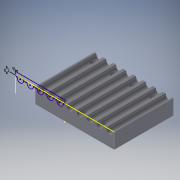
# Autodesk Inventor part: belt-clamp-15mm-htd
Saved by Autodesk Inventor 2016 (Build 200138000, 138)
## iProperties
Created: 2015-10-25
Part Number: belt-clamp-15mm-htd
Material: Generic
Document SubType Name: Modeling
Designer: as
Density: 1 g/cm^3
Appearance: Default
Author: as
Autodesk Inventor part; units mm, degrees
ref_plane "YZ Plane" through (0, 0, 0) normal (1, 0, 0) x (0, 1, 0)
ref_plane "XZ Plane" through (0, 0, 0) normal (0, 1, 0) x (-1, 0, 0)
ref_plane "XY Plane" through (0, 0, 0) normal (0, 0, 1) x (1, 0, 0)
sketch "HTD 5m profile" plane through (0, 0, 0) normal (0, 0, 1) x (1, 0, 0)
  arc A0 (5.5026, 4.809) -> (5.0726, 4.379) centre (5.5026, 4.379) ccw
  line L0 (5.0726, 4.379) -> (5.0726, 4.229)
  arc A1 (3.5726, 2.729) -> (5.0726, 4.229) centre (3.5726, 4.229) ccw
  line L1 (3.5726, 2.729) -> (3.4726, 2.729)
  arc A2 (1.9726, 4.229) -> (3.4726, 2.729) centre (3.4726, 4.229) ccw
  line L2 (1.9726, 4.229) -> (1.9726, 4.379)
  arc A3 (1.9726, 4.379) -> (1.5426, 4.809) centre (1.5426, 4.379) ccw
  line L3 (1.5426, 4.809) -> (0.9326, 4.809)
  line L4 (0.9326, 4.809) -> (0.9326, 6.539)
  line L5 (6.5426, 4.809) -> (5.5026, 4.809)
  arc A4 (10.5026, 4.809) -> (10.0726, 4.379) centre (10.5026, 4.379) ccw
  line L6 (10.0726, 4.379) -> (10.0726, 4.229)
  arc A5 (8.5726, 2.729) -> (10.0726, 4.229) centre (8.5726, 4.229) ccw
  line L7 (8.5726, 2.729) -> (8.4726, 2.729)
  arc A6 (6.9726, 4.229) -> (8.4726, 2.729) centre (8.4726, 4.229) ccw
  line L8 (6.9726, 4.229) -> (6.9726, 4.379)
  arc A7 (6.9726, 4.379) -> (6.5426, 4.809) centre (6.5426, 4.379) ccw
  line L9 (11.5426, 4.809) -> (10.5026, 4.809)
  arc A8 (15.5026, 4.809) -> (15.0726, 4.379) centre (15.5026, 4.379) ccw
  line L10 (15.0726, 4.379) -> (15.0726, 4.229)
  arc A9 (13.5726, 2.729) -> (15.0726, 4.229) centre (13.5726, 4.229) ccw
  line L11 (13.5726, 2.729) -> (13.4726, 2.729)
  arc A10 (11.9726, 4.229) -> (13.4726, 2.729) centre (13.4726, 4.229) ccw
  line L12 (11.9726, 4.229) -> (11.9726, 4.379)
  arc A11 (11.9726, 4.379) -> (11.5426, 4.809) centre (11.5426, 4.379) ccw
  line L13 (16.5426, 4.809) -> (15.5026, 4.809)
  arc A12 (20.5026, 4.809) -> (20.0726, 4.379) centre (20.5026, 4.379) ccw
  line L14 (20.0726, 4.379) -> (20.0726, 4.229)
  arc A13 (18.5726, 2.729) -> (20.0726, 4.229) centre (18.5726, 4.229) ccw
  line L15 (18.5726, 2.729) -> (18.4726, 2.729)
  arc A14 (16.9726, 4.229) -> (18.4726, 2.729) centre (18.4726, 4.229) ccw
  line L16 (16.9726, 4.229) -> (16.9726, 4.379)
  arc A15 (16.9726, 4.379) -> (16.5426, 4.809) centre (16.5426, 4.379) ccw
  line L17 (21.5426, 4.809) -> (20.5026, 4.809)
  line L18 (26.1126, 4.809) -> (25.5026, 4.809)
  arc A16 (25.5026, 4.809) -> (25.0726, 4.379) centre (25.5026, 4.379) ccw
  line L19 (25.0726, 4.379) -> (25.0726, 4.229)
  arc A17 (23.5726, 2.729) -> (25.0726, 4.229) centre (23.5726, 4.229) ccw
  line L20 (23.5726, 2.729) -> (23.4726, 2.729)
  arc A18 (21.9726, 4.229) -> (23.4726, 2.729) centre (23.4726, 4.229) ccw
  line L21 (21.9726, 4.229) -> (21.9726, 4.379)
  arc A19 (21.9726, 4.379) -> (21.5426, 4.809) centre (21.5426, 4.379) ccw
  line L22 (0.9326, 6.539) -> (26.1126, 6.539)
  line L23 (26.1126, 6.539) -> (26.1126, 4.809)
  point P0 (13.5226, 4.1974)
sketch "Sketch1" plane through (0, 0, 0) normal (0, 0, 1) x (1, 0, 0)
  line L0 (25, 15) -> (-25, 15)
  line L1 (-25, 15) -> (-25, -15)
  line L2 (-25, -15) -> (25, -15)
  line L3 (25, -15) -> (25, 15)
  line L4 (25, 15) -> (-25, -15) construction
  line L5 (-25, 15) -> (25, -15) construction
  point P0 (0, 0)
  dimension "d0" = 50
  dimension "d1" = 30
  constraints: 12 end point, 2 midpoint, 2 parallel, 1 horizontal, 1 perpendicular
  measures "d0" distance of L2.end L1.end
  measures "d1" distance of L1.end L0.end
extrude "Extrusion1" add sketch "Sketch1" along normal blind 8
sketch "Sketch2" plane through (-25, -15, 0) normal (0, -1, 0) x (1, 0, 0)
  line L0 (0, 8) -> (50, 8) projected
  line L1 (0, 0) -> (0, 8) projected
  arc A0 (4.57, 7.8) -> (4.14, 7.37) centre (4.57, 7.37) ccw
  line L2 (4.14, 7.37) -> (4.14, 7.22)
  arc A1 (2.64, 5.72) -> (4.14, 7.22) centre (2.64, 7.22) ccw
  line L3 (2.64, 5.72) -> (2.54, 5.72)
  arc A2 (1.04, 7.22) -> (2.54, 5.72) centre (2.54, 7.22) ccw
  line L4 (1.04, 7.22) -> (1.04, 7.37)
  arc A3 (1.04, 7.37) -> (0.61, 7.8) centre (0.61, 7.37) ccw
  line L5 (0.61, 7.8) -> (0, 7.8)
  line L6 (0, 7.8) -> (0, 9.53)
  line L7 (5.61, 7.8) -> (4.57, 7.8)
  arc A4 (9.57, 7.8) -> (9.14, 7.37) centre (9.57, 7.37) ccw
  line L8 (9.14, 7.37) -> (9.14, 7.22)
  arc A5 (7.64, 5.72) -> (9.14, 7.22) centre (7.64, 7.22) ccw
  line L9 (7.64, 5.72) -> (7.54, 5.72)
  arc A6 (6.04, 7.22) -> (7.54, 5.72) centre (7.54, 7.22) ccw
  line L10 (6.04, 7.22) -> (6.04, 7.37)
  arc A7 (6.04, 7.37) -> (5.61, 7.8) centre (5.61, 7.37) ccw
  line L11 (10.61, 7.8) -> (9.57, 7.8)
  arc A8 (14.57, 7.8) -> (14.14, 7.37) centre (14.57, 7.37) ccw
  line L12 (14.14, 7.37) -> (14.14, 7.22)
  arc A9 (12.64, 5.72) -> (14.14, 7.22) centre (12.64, 7.22) ccw
  line L13 (12.64, 5.72) -> (12.54, 5.72)
  arc A10 (11.04, 7.22) -> (12.54, 5.72) centre (12.54, 7.22) ccw
  line L14 (11.04, 7.22) -> (11.04, 7.37)
  arc A11 (11.04, 7.37) -> (10.61, 7.8) centre (10.61, 7.37) ccw
  line L15 (15.61, 7.8) -> (14.57, 7.8)
  arc A12 (19.57, 7.8) -> (19.14, 7.37) centre (19.57, 7.37) ccw
  line L16 (19.14, 7.37) -> (19.14, 7.22)
  arc A13 (17.64, 5.72) -> (19.14, 7.22) centre (17.64, 7.22) ccw
  line L17 (17.64, 5.72) -> (17.54, 5.72)
  arc A14 (16.04, 7.22) -> (17.54, 5.72) centre (17.54, 7.22) ccw
  line L18 (16.04, 7.22) -> (16.04, 7.37)
  arc A15 (16.04, 7.37) -> (15.61, 7.8) centre (15.61, 7.37) ccw
  line L19 (20.61, 7.8) -> (19.57, 7.8)
  line L20 (25.18, 7.8) -> (24.57, 7.8)
  arc A16 (24.57, 7.8) -> (24.14, 7.37) centre (24.57, 7.37) ccw
  line L21 (24.14, 7.37) -> (24.14, 7.22)
  arc A17 (22.64, 5.72) -> (24.14, 7.22) centre (22.64, 7.22) ccw
  line L22 (22.64, 5.72) -> (22.54, 5.72)
  arc A18 (21.04, 7.22) -> (22.54, 5.72) centre (22.54, 7.22) ccw
  line L23 (21.04, 7.22) -> (21.04, 7.37)
  arc A19 (21.04, 7.37) -> (20.61, 7.8) centre (20.61, 7.37) ccw
  line L24 (0, 9.53) -> (25.18, 9.53)
  line L25 (25.18, 9.53) -> (25.18, 7.8)
  point P0 (25, 0)
  dimension "d4" = 0.2
  dimension "d9" = 0
  constraints: 1 horizontal
  measures "d9" horizontal extent of L1
sketch "Sketch3" plane through (-25, -15, 0) normal (0, -1, 0) x (1, 0, 0)
  line L0 (10.61, 7.8) -> (9.57, 7.8) projected
  line L1 (5.61, 7.8) -> (4.57, 7.8) projected
  arc A0 (6.04, 7.22) -> (7.54, 5.72) centre (7.54, 7.22) ccw projected
  arc A1 (6.04, 7.37) -> (5.61, 7.8) centre (5.61, 7.37) ccw projected
  arc A2 (9.57, 7.8) -> (9.14, 7.37) centre (9.57, 7.37) ccw projected
  circle A3 centre (9.4887, 5.42) radius 1.5
  arc A4 (9.57, 7.8) -> (9.14, 7.37) centre (9.57, 7.37) ccw
  arc A5 (6.04, 7.37) -> (5.61, 7.8) centre (5.61, 7.37) ccw
  line L2 (4.57, 7.8) -> (5.61, 7.8)
  line L3 (9.57, 7.8) -> (10.61, 7.8)
  arc A6 (7.64, 5.72) -> (9.14, 7.37) centre (7.4825, 7.37) ccw
  arc A7 (6.04, 7.37) -> (7.64, 5.72) centre (7.6908, 7.37) ccw
  line L4 (5.61, 7.8) -> (5.61, 8.8)
  line L5 (10.61, 7.8) -> (10.61, 8.8)
  line L6 (10.61, 8.8) -> (5.61, 8.8)
  point P0 (25, 0)
  point P1 (4.57, 7.37)
  point P2 (5.61, 7.37)
  point P3 (7.54, 7.22)
  point P4 (7.64, 7.22)
  point P5 (9.57, 7.37)
  point P6 (10.61, 7.37)
  dimension "d5" = 1
  dimension "d6" = 1
  constraints: 11 end point, 8 point on circle, 5 centre point, 4 tangent, 3 coincident, 2 collinear, 1 concentric, 1 perpendicular, 1 vertical
  measures "d5" distance of L2.end L4.end
  measures "d6" distance of L0.start L5.end
extrude "Extrusion2" cut sketch "Sketch3" against normal through all contours L0 A2 A6 A3 A7 A1 L4 L6 L5 | A6 A3 picked at (8.4541, 6.1804)
pattern_linear "Rectangular Pattern1" count 10 spacing 5 along (1, 0, 0) of "Extrusion2"
sketch "Sketch4" plane through (0, 0, 0) normal (0, 0, -1) x (-1, 0, 0)
  line L0 (-25, -15) -> (-25, 15) construction
  line L1 (25, 12) -> (-25, 12) construction
  line L2 (-25, 12) -> (-25, -12) construction
  line L3 (-25, -12) -> (25, -12) construction
  line L4 (25, -12) -> (25, 12) construction
  line L5 (25, 12) -> (-25, -12) construction
  line L6 (-25, 12) -> (25, -12) construction
  line L7 (32.7257, -12) -> (-34.362, -12) construction
  line L8 (25, 15) -> (25, -15) projected
  point P0 (0, 0)
  point P1 (22.5, -12)
  dimension "d13" = 24
  dimension "d14" = 0
  dimension "d15" = 2.5
  constraints: 14 end point, 2 horizontal, 2 midpoint, 2 parallel, 2 point on line, 1 perpendicular
  measures "d13" distance of L2.end L1.end
  measures "d14" distance between parallel lines of L3 L7
  measures "d15" distance from line of L8 point (22.5, -12)
hole "Hole1" at (-22.5, -12, 0) direction (0, 0, 1) diameter 2.459 end through all thread size "M3x0.5" class "6H" standard "ISO Metric profile"
pattern_linear "Rectangular Pattern2" count 5 spacing 10 along (1, 0, 0) count 2 spacing 24 along (0, 1, 0) of "Hole1"
move faces "Move1" translate (10, 0, 0) faces at (-25, 5, 2.6667)
chamfer "Chamfer1" distance 0.25 angle 45 8 edges at (5, 15, 0) (25, 0, 0) (5, -15, 0) (-15, 0, 0) (25, 15, 3.9) (25, -15, 3.9) (-15, 15, 3.9) (-15, -15, 3.9)
body "Solid1"
